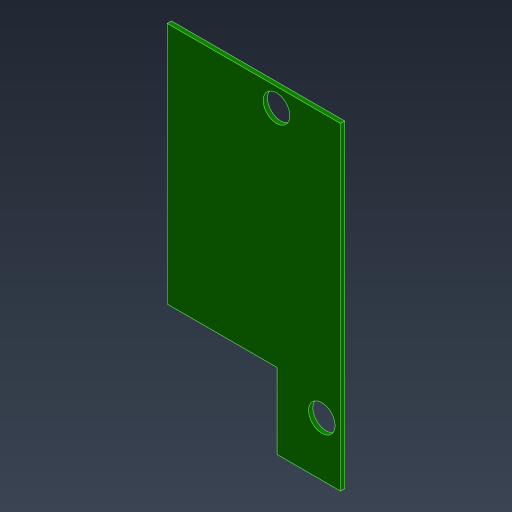
# Autodesk Inventor part: PCB-INTERFACE-dummy
Saved by Autodesk Inventor 2023 (Build 270158000, 158)
## iProperties
Created: 2025-04-11
Part Number: PCB-INTERFACE-dummy
Material: Generic
Document SubType Name: Modeling
Designer: szymo
Density: 1 g/cm^3
Appearance: Default(1)
Mass: 1.65788 g
Surface Area: 35.2189 cm^2
Volume: 1.65788 cm^3
Author: szymo
Autodesk Inventor part; units mm, degrees
ref_plane "YZ Plane" through (0, 0, 0) normal (1, 0, 0) x (0, 1, 0)
ref_plane "XZ Plane" through (0, 0, 0) normal (0, 1, 0) x (-1, 0, 0)
ref_plane "XY Plane" through (0, 0, 0) normal (0, 0, 1) x (1, 0, 0)
sketch "Sketch1" plane through (0, 0, 0) normal (0, 0, 1) x (1, 0, 0)
  circle A0 centre (29.1588, -35.9) radius 2.5 projected
  line L0 (20.2762, -32.4) -> (32.6588, -32.4) projected
  line L1 (20.2762, -32.4) -> (20.2762, -46) projected
  line L2 (32.6588, -46) -> (20.2762, -46) projected
  line L3 (32.6588, -32.4) -> (32.6588, -46) projected
  circle A1 centre (-11.075, -42.75) radius 2.5 projected
  line L4 (-2.7317, -32.4) -> (10.1583, -32.4) projected
  line L5 (-2.7317, -32.4) -> (-2.7317, -37.7) projected
  line L6 (-2.7317, -37.7) -> (-21.3412, -37.7) projected
  line L7 (-21.3412, -37.7) -> (-21.3412, -46) projected
  line L8 (10.1583, -46) -> (-21.3412, -46) projected
  line L9 (10.1583, -32.4) -> (10.1583, -46) projected
  circle A2 centre (20.672, 10.1) radius 2.5 projected
  line L10 (-0.2933, 0) -> (12.6492, 0) projected
  line L11 (12.6492, 0) -> (12.6492, 5.3) projected
  line L12 (12.6492, 5.3) -> (32.6588, 5.3) projected
  line L13 (32.6588, 5.3) -> (32.6588, 13.6) projected
  line L14 (-0.2933, 13.6) -> (32.6588, 13.6) projected
  line L15 (-0.2933, 0) -> (-0.2933, 13.6) projected
  circle A3 centre (-17.3412, 4) radius 2.5 projected
  line L16 (-21.3412, 0) -> (-10.5199, 0) projected
  line L17 (-10.5199, 0) -> (-10.5199, 13.6) projected
  line L18 (-21.3412, 13.6) -> (-10.5199, 13.6) projected
  line L19 (-21.3412, 0) -> (-21.3412, 13.6) projected
  circle A4 centre (20.672, 10.1) radius 1.8
  circle A5 centre (29.1588, -35.9) radius 1.8
  line L20 (20.7762, -46) -> (20.7762, -31.9)
  line L21 (20.7762, -31.9) -> (0.2067, -31.9)
  line L22 (0.2067, -31.9) -> (0.2067, 13.6)
  line L23 (32.6588, 13.6) -> (32.6588, -46)
  dimension "d17" = 3.6
  dimension "d18" = 3.6
  dimension "d19" = 0.5
  dimension "d20" = 0.5
  dimension "d21" = 0.5
  constraints: 8 end point, 3 perpendicular, 2 centre point, 2 coincident, 2 point on line, 1 vertical
  measures "d17" diameter of A4
  measures "d18" diameter of A5
  measures "d19" distance between parallel lines of L15 L22
  measures "d20" distance between parallel lines of L1 L20
  measures "d21" distance from line of L21 L0.start
extrude "Extrusion1" add sketch "Sketch1" along normal blind 0.8 contours L20 L21 L22 L10 L11 L12 L23 L0 | L0 L3 L2 L20 | L12 L11 L10 L22 L14 L13
body "Solid1"
